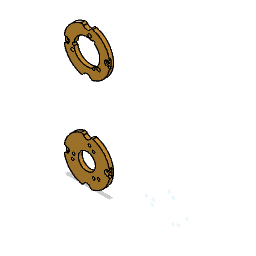
SlipRing_Mount v1.2 (Autodesk Fusion 360 design; units mm, degrees)
Autodesk Fusion 360 part; units mm, degrees
note: some values were not read from the file. Set by a fixed rule: which face or edge a step refers to.
sketch "Sketch1" plane through (0, 0, 0) normal (0, 0, 1) x (1, 0, 0)
  circle A0 centre (0, 0) radius 30
  dimension "d1" = 60
  constraint coincident A0.centre origin
  measures "d1" diameter of A0
extrude "Extrude1" add sketch "Sketch1" along normal blind 3 makes body 1
sketch "Sketch2" plane through (0, 0, 3) normal (0, 0, 1) x (1, 0, 0)
  circle A0 centre (0, 0) radius 30
  circle A1 centre (0, 0) radius 12
  dimension "d4" = 24
  constraint concentric A0 A1
  measures "d4" diameter of A1
extrude "Extrude2" cut sketch "Sketch2" against normal blind 5 contours A1 bodies 1
sketch "Sketch3" plane through (0, 0, 3) normal (0, 0, 1) x (1, 0, 0)
  circle A0 centre (0, 0) radius 12
  circle A1 centre (0, 0) radius 30
  circle A2 centre (26.7, 0.0327) radius 2
  circle A3 centre (-26.7, 0.0326) radius 2
  dimension "d8" = 4
  dimension "d9" = 4
  measures "d8" diameter of A2
  measures "d9" diameter of A3
extrude "Extrude3" cut sketch "Sketch3" against normal blind 5 contours A2 | A3 bodies 1
sketch "Sketch4" plane through (0, 0, 3) normal (0, 0, 1) x (1, 0, 0)
  circle A0 centre (26.7, 0.0327) radius 2
  circle A1 centre (-26.7, 0.0326) radius 2
  circle A2 centre (0, 0) radius 12
  circle A3 centre (0, 0) radius 30
  circle A4 centre (0, 0) radius 12
  line L0 (0, 0) -> (20, 0) construction
  line L1 (0, 0) -> (20, 0) construction
  line L2 (0, 0) -> (20, 0) construction
  circle A5 centre (3.473, 19.6962) radius 1.75
  circle A6 centre (-18.7939, -6.8404) radius 1.75
  circle A7 centre (15.3209, -12.8558) radius 1.75
  line L3 (0, 0) -> (17.5, 0) construction
  circle A8 centre (8.75, 15.1554) radius 1.75
  circle A9 centre (8.75, -15.1554) radius 1.75
  circle A10 centre (-17.5, 0) radius 1.75
  line L4 (0, 0) -> (12, 0) construction
  circle A11 centre (10.3923, -6) radius 1.75
  circle A12 centre (0, 12) radius 1.75
  circle A13 centre (-10.3923, -6) radius 1.75
  dimension "d24" = 3.5
  dimension "d26" = 3.5
  dimension "d27" = 3.5
  dimension "d30" = 3.5
  dimension "d31" = 3.5
  dimension "d32" = 3.5
  dimension "d35" = 3.5
  dimension "d36" = 3.5
  dimension "d37" = 3.5
  constraint coincident A2.centre A3.centre
  constraint horizontal L0
  constraint horizontal L1
  constraint horizontal L2
  constraint horizontal L3
  constraint horizontal L4
  measures "d24" diameter of A5
  measures "d26" diameter of A6
  measures "d27" diameter of A7
  measures "d30" diameter of A8
  measures "d31" diameter of A9
  measures "d32" diameter of A10
  measures "d35" diameter of A11
  measures "d36" diameter of A12
  measures "d37" diameter of A13
extrude "Extrude4" cut sketch "Sketch4" against normal blind 16 contours A2 A4 A12 | A2 A4 A11 | A2 A4 A13 | A5 | A6 | A7 | A8 | A9 | A10 picked at (-0.0213, 12.5735) picked at (10.8727, -6.314) picked at (-10.8893, -6.2869) bodies 1
extrude "Extrude5" add 1 faces at (21.0883, 6.6262, 3) along direction (0, 0, 1) blind 2 on bodies 1 bodies 1
copy_body "Körper kopieren/einfügen1" bodies 1 makes body 2
move_body "Verschieben1" bodies 2 to x (1, 0, 0) y (0, 1, 0) z (0, 0, 1) at (105.0375, 0, 0)
ref_plane "Arbeitsebene1" through (105.0375, 0, 0) normal (0, 0, -1) x (-1, 0, 0)
sketch "Skizze5" plane through (105.0375, 0, 0) normal (0, 0, -1) x (1, 0, 0)
delete_face "Fläche löschen1" 2 faces at (94.2119, -7.6955, 4.3333) (94.2119, -7.6955, 1) on bodies 2
delete_face "Fläche löschen2" 2 faces at (115.8631, -7.6955, 3.6667) (115.7782, -7.715, 2) on bodies 2
delete_face "Fläche löschen3" 2 faces at (105.8736, 13.5373, 3.6667) (104.1259, 13.4938, 1) on bodies 2
move_face "Flächen versetzen1" offset 5 3 faces at (115.1404, -6.4755, 2.6667) (114.0925, -7.8745, 1) (113.719, -8.2844, 3.6667) on bodies 2
move_face "Flächen versetzen2" offset 0.8 4 faces at (-24.7025, -0.0671, 4.3333) (-24.7099, -0.1666, 2) (28.6975, -0.067, 4.3333) (28.69, -0.1664, 2) on bodies 1
delete_face "Fläche löschen4" 2 faces at (-11.3074, -4.5083, 4.3333) (-11.3074, -4.5083, 1) on bodies 1
delete_face "Fläche löschen5" 2 faces at (10.8256, -7.6955, 4.3333) (11.3074, -4.5083, 1) on bodies 1
delete_face "Fläche löschen6" 2 faces at (-1.7494, 12.0466, 3.6667) (-1.7494, 12.0466, 2) on bodies 1
move_face "Flächen versetzen3" offset 0.8 3 faces at (10.1029, -6.4755, 2.6667) (8.6815, -8.2844, 2) (8.6815, -8.2844, 3.6667) on bodies 1
sketch "Sketch6" plane through (0, 0, 5) normal (0, 0, 1) x (1, 0, 0)
  circle A0 centre (-17.5, 0) radius 1.75
  circle A1 centre (-18.7939, -6.8404) radius 1.75
  circle A2 centre (3.473, 19.6962) radius 1.75
  circle A3 centre (8.75, -15.1554) radius 1.75
  circle A4 centre (15.3209, -12.8558) radius 1.75
  circle A5 centre (8.75, 15.1554) radius 1.75
  circle A6 centre (26.7, 0.0327) radius 1.2
  circle A7 centre (-26.7, 0.0326) radius 1.2
  circle A8 centre (0, 0) radius 11.2
  circle A9 centre (0, 0) radius 30
  circle A10 centre (-0.0183, 30) radius 5
  circle A11 centre (-0.0119, -30) radius 5
  dimension "d46" = 10
  dimension "d47" = 10
  constraint coincident A9 A10.centre
  constraint coincident A9 A11.centre
  measures "d46" diameter of A10
  measures "d47" diameter of A11
extrude "Extrude6" cut sketch "Sketch6" against normal blind 8 contours A9 A10 | A9 A11 picked at (-0.0173, 28.3024) picked at (-0.0112, -28.3024) bodies 1
fillet "Fillet1" radius 3 2 edges at (4.9646, 29.5864, 2.5) (-5.0007, 29.5803, 2.5) on bodies 1
fillet "Fillet2" radius 3 2 edges at (-4.9943, -29.5814, 2.5) (4.9709, -29.5853, 2.5) on bodies 1
move_face "OffsetFaces4" offset 0.5 2 faces at (77.0142, 1.5321, 2) (77.0142, 1.5321, 3.6667) on bodies 2
move_face "OffsetFaces5" offset 0.5 2 faces at (130.8251, -1.747, 1) (130.9149, 1.8557, 4.3333) on bodies 2
sketch "Sketch7" plane through (0, 0, 5) normal (0, 0, 1) x (1, 0, 0)
  circle A0 centre (87.5375, 0) radius 1.75
  circle A1 centre (86.2437, -6.8404) radius 1.75
  circle A2 centre (108.5105, 19.6962) radius 1.75
  circle A3 centre (113.7875, -15.1554) radius 1.75
  circle A4 centre (120.3584, -12.8558) radius 1.75
  circle A5 centre (113.7875, 15.1554) radius 1.75
  circle A6 centre (131.7375, 0.0327) radius 1.5
  circle A7 centre (78.3375, 0.0326) radius 1.5
move_face "OffsetFaces6" offset 2 3 faces at (110.9309, -3.7774, 2.6667) (102.3578, -6.4668, 1) (99.9733, -4.8326, 4.3333) on bodies 2
sketch "Sketch8" plane through (0, 0, 5) normal (0, 0, 1) x (1, 0, 0)
sketch "Sketch9" plane through (0, 0, 5) normal (0, 0, 1) x (1, 0, 0)
  circle A0 centre (106.4956, 8.6212) radius 1.75
  circle A1 centre (96.7895, -3.0249) radius 1.75
  circle A2 centre (111.7042, -5.6229) radius 1.75
  dimension "d59" = 3.5
  dimension "d61" = 3.5
  dimension "d62" = 3.5
  measures "d59" diameter of A0
  measures "d61" diameter of A1
  measures "d62" diameter of A2
extrude "Extrude7" cut sketch "Sketch9" against normal blind 15 bodies 2
sketch "Sketch10" plane through (0, 0, 5) normal (0, 0, 1) x (1, 0, 0)
  circle A0 centre (105.0021, 0.0015) radius 28.0015
  circle A1 centre (104.9996, 28.0029) radius 4
  circle A2 centre (105, -28) radius 4
  dimension "d65" = 8
  constraint coincident A0 A1.centre
  constraint coincident A0 A2.centre
  measures "d65" diameter of A2
extrude "Extrude8" cut sketch "Sketch10" against normal blind 15 contours A0 A1 | A0 A1 | A0 A2 | A0 A2 bodies 2
fillet "Fillet3" radius 2 2 edges at (101.4164, 29.7807, 2.5) (108.5781, 29.7903, 2.5) on bodies 2
fillet "Fillet4" radius 2 2 edges at (101.4183, -29.7809, 2.5) (108.5769, -29.7905, 2.5) on bodies 2
copy_body "CopyPasteBodies2" bodies 1 makes body 3
move_body "Move2" bodies 3 to x (1, 0, 0) y (0, 1, 0) z (0, 0, 1) at (0, 125, 0)
sketch "Sketch11" plane through (0, 0, 5) normal (0, 0, 1) x (1, 0, 0)
  arc A0 (4.3489, 97.4462) -> (7.7393, 96.0155) centre (6.9653, 98.9139) ccw
  arc A1 (7.7393, 96.0155) -> (7.733, 153.9862) centre (0, 125) ccw
  arc A2 (7.733, 153.9862) -> (4.343, 152.5547) centre (6.9597, 151.0876) ccw
  arc A3 (-4.3766, 152.5494) -> (4.343, 152.5547) centre (-0.0183, 155) ccw
  arc A4 (-4.3766, 152.5494) -> (-7.7684, 153.9767) centre (-6.9916, 151.0791) ccw
  arc A5 (-7.7684, 153.9767) -> (-7.7622, 96.0216) centre (0, 125) ccw
  arc A6 (-7.7622, 96.0216) -> (-4.3707, 97.4496) centre (-6.986, 98.9194) ccw
  arc A7 (4.3489, 97.4462) -> (-4.3707, 97.4496) centre (-0.0119, 95) ccw
  circle A8 centre (0, 125) radius 11.2
  circle A9 centre (-26.7, 125.0326) radius 1.2
  circle A10 centre (26.7, 125.0327) radius 1.2
  circle A11 centre (8.75, 140.1554) radius 1.75
  circle A12 centre (15.3209, 112.1442) radius 1.75
  circle A13 centre (8.75, 109.8446) radius 1.75
  circle A14 centre (3.473, 144.6962) radius 1.75
  circle A15 centre (-18.7939, 118.1596) radius 1.75
  circle A16 centre (-17.5, 125) radius 1.75
  circle A17 centre (0, 125) radius 17
  dimension "d72" = 34
  constraint concentric A1 A17
  measures "d72" diameter of A17
extrude "Extrude9" cut sketch "Sketch11" against normal blind 5 contours A11 A13 A16 A17 bodies 3
move_face "OffsetFaces7" offset -0.5 3 faces at (-20.4064, 117.4798, 3.3333) (1.9361, 145.5331, 3.3333) (16.9654, 112.7428, 1.6667) on bodies 3
sketch "Sketch12" plane through (0, 0, 5) normal (0, 0, 1) x (1, 0, 0)
  circle A0 centre (-18.7939, 118.1596) radius 2.25
  circle A1 centre (3.473, 144.6962) radius 2.25
  circle A2 centre (15.3209, 112.1442) radius 2.25
  arc A3 (-16.9196, 123.349) -> (7.03, 109.5217) centre (0, 125) ccw
  arc A4 (-16.9196, 126.651) -> (-16.9196, 123.349) centre (-17.5, 125) ccw
  arc A5 (7.03, 140.4783) -> (-16.9196, 126.651) centre (0, 125) ccw
  arc A6 (9.8896, 138.8274) -> (7.03, 140.4783) centre (8.75, 140.1554) ccw
  arc A7 (9.8896, 111.1726) -> (9.8896, 138.8274) centre (0, 125) ccw
  arc A8 (7.03, 109.5217) -> (9.8896, 111.1726) centre (8.75, 109.8446) ccw
  circle A9 centre (26.7, 125.0327) radius 1.2
  circle A10 centre (-26.7, 125.0326) radius 1.2
  arc A11 (4.3489, 97.4462) -> (7.7393, 96.0155) centre (6.9653, 98.9139) ccw
  arc A12 (7.7393, 96.0155) -> (7.733, 153.9862) centre (0, 125) ccw
  arc A13 (7.733, 153.9862) -> (4.343, 152.5547) centre (6.9597, 151.0876) ccw
  arc A14 (-4.3766, 152.5494) -> (4.343, 152.5547) centre (-0.0183, 155) ccw
  arc A15 (-4.3766, 152.5494) -> (-7.7684, 153.9767) centre (-6.9916, 151.0791) ccw
  arc A16 (-7.7684, 153.9767) -> (-7.7622, 96.0216) centre (0, 125) ccw
  arc A17 (-7.7622, 96.0216) -> (-4.3707, 97.4496) centre (-6.986, 98.9194) ccw
  arc A18 (4.3489, 97.4462) -> (-4.3707, 97.4496) centre (-0.0119, 95) ccw
  circle A19 centre (26.7, 125.0327) radius 3.5
  circle A20 centre (-26.7, 125.0326) radius 3.5
  dimension "d76" = 7
  dimension "d77" = 7
  constraint concentric A9 A19
  constraint concentric A10 A20
  measures "d76" diameter of A19
  measures "d77" diameter of A20
extrude "Extrude10" cut sketch "Sketch12" against normal blind 2 contours A12 A19 | A16 A20 picked at (29.2981, 125.0354) picked at (-29.2981, 125.0352) bodies 3
fillet "Fillet5" radius 2 4 edges at (29.976, 123.8008, 4) (29.973, 126.2726, 4) (-29.976, 123.8007, 4) (-29.973, 126.2725, 4) on bodies 3
sketch "Sketch13" plane through (0, 0, 5) normal (0, 0, 1) x (1, 0, 0)
  arc A0 (4.3489, -27.5538) -> (7.7393, -28.9845) centre (6.9653, -26.0861) ccw
  arc A1 (7.7393, -28.9845) -> (7.733, 28.9862) centre (0, 0) ccw
  arc A2 (7.733, 28.9862) -> (4.343, 27.5547) centre (6.9597, 26.0876) ccw
  arc A3 (-4.3766, 27.5494) -> (4.343, 27.5547) centre (-0.0183, 30) ccw
  arc A4 (-4.3766, 27.5494) -> (-7.7684, 28.9767) centre (-6.9916, 26.0791) ccw
  arc A5 (-7.7684, 28.9767) -> (-7.7622, -28.9784) centre (0, 0) ccw
  arc A6 (-7.7622, -28.9784) -> (-4.3707, -27.5504) centre (-6.986, -26.0806) ccw
  arc A7 (4.3489, -27.5538) -> (-4.3707, -27.5504) centre (-0.0119, -30) ccw
  circle A8 centre (0, 0) radius 11.2
  circle A9 centre (-26.7, 0.0326) radius 1.2
  circle A10 centre (26.7, 0.0327) radius 1.2
  circle A11 centre (8.75, 15.1554) radius 1.75
  circle A12 centre (15.3209, -12.8558) radius 1.75
  circle A13 centre (8.75, -15.1554) radius 1.75
  circle A14 centre (3.473, 19.6962) radius 1.75
  circle A15 centre (-18.7939, -6.8404) radius 1.75
  circle A16 centre (-17.5, 0) radius 1.75
  circle A17 centre (26.7, 0.0327) radius 3.5
  circle A18 centre (-26.7, 0.0326) radius 3.5
  dimension "d82" = 7
  dimension "d83" = 7
  constraint concentric A10 A17
  constraint concentric A9 A18
  measures "d82" diameter of A17
  measures "d83" diameter of A18
extrude "Extrude11" cut sketch "Sketch13" against normal blind 3 contours A1 A17 | A1 A17 | A5 A18 | A5 A18 bodies 1
fillet "Fillet6" radius 2 2 edges at (29.973, 1.2726, 3.5) (29.976, -1.1992, 3.5) on bodies 1
fillet "Fillet7" radius 2 2 edges at (-29.976, -1.1993, 3.5) (-29.973, 1.2725, 3.5) on bodies 1
hidden bodies 2
named bodies: "Com_SlipRing_stage", "SlipRing_stage", "SlipRing_stage (1)", "Com_SlipRing_stage for Ephys+Miniscope"
